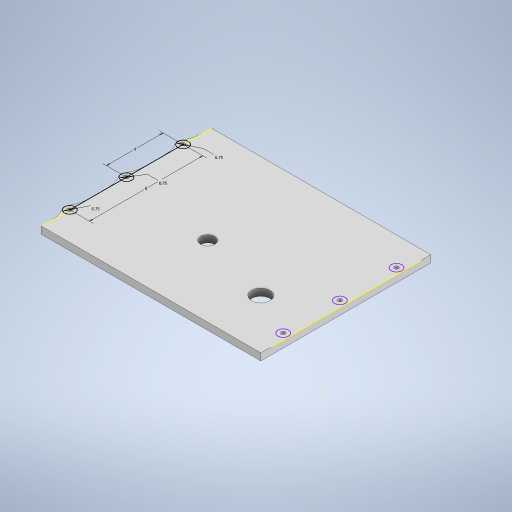
# Autodesk Inventor part: chassis_cap
Saved by Autodesk Inventor 2023 (Build 270158000, 158)
## iProperties
Created: 2023-05-04
Part Number: chassis_cap
Material: Generic
Document SubType Name: Modeling
Designer: user
Density: 1 g/cm^3
Appearance: Default
Author: user
Autodesk Inventor part; units mm, degrees
ref_plane "YZ Plane" through (0, 0, 0) normal (1, 0, 0) x (0, 1, 0)
ref_plane "XZ Plane" through (0, 0, 0) normal (0, 1, 0) x (-1, 0, 0)
ref_plane "XY Plane" through (0, 0, 0) normal (0, 0, 1) x (1, 0, 0)
sketch "Sketch2" plane through (0, 0, 0) normal (0, 1, 0) x (-1, 0, 0)
  line L0 (0, 0) -> (200, 0)
  line L1 (200, 0) -> (200, -120)
  line L2 (200, -120) -> (0, -120)
  line L3 (0, -120) -> (0, 0)
  dimension "d0" = 200
  dimension "d1" = 120
  constraints: 8 end point, 2 parallel, 1 horizontal, 1 perpendicular
  measures "d0" distance of L1.end L2.end
  measures "d1" distance of L0.end L1.end
extrude "Extrusion1" add sketch "Sketch2" along normal blind 50
sketch "Sketch3" plane through (0, 50, 0) normal (0, 1, 0) x (1, 0, 0)
  line L0 (0, 120) -> (-200, 120) projected
  line L1 (0, 120) -> (0, 113)
  line L2 (0, 0) -> (0, 120) projected
  line L3 (-200, 0) -> (0, 0) projected
  line L4 (0, 0) -> (0, 7)
  line L5 (0, 7) -> (-45, 7)
  line L6 (-45, 7) -> (-45, 113)
  line L7 (-45, 113) -> (0, 113)
  line L8 (0, 113) -> (0, 7)
  dimension "d4" = 7
  dimension "d5" = 7
  dimension "d6" = 45
  constraints: 12 end point, 2 parallel, 2 point on line, 1 horizontal, 1 perpendicular
  measures "d4" distance of L0.start L1.end
  measures "d5" distance of L2.start L4.end
  measures "d6" distance of L6.end L7.end
extrude "Extrusion2" cut sketch "Sketch3" against normal blind 50
sketch "Sketch6" plane through (-200, 0, 0) normal (0, 0, 1) x (1, 0, 0)
  line L0 (200, 0) -> (200, 50) projected
  line L1 (200, 0) -> (205, 0)
  line L2 (205, 0) -> (205, 50)
  line L3 (205, 50) -> (200, 50)
  line L4 (200, 50) -> (200, 0)
  dimension "d42" = 5
  constraints: 8 end point, 2 parallel, 1 horizontal, 1 perpendicular
  measures "d42" distance of L3.end L2.end
extrude "Extrusion4" add sketch "Sketch6" against normal blind 7
sketch "Sketch7" plane through (0, 0, -120) normal (0, 0, -1) x (-1, 0, 0)
  line L0 (45, 50) -> (0, 50) projected
  line L1 (200, 0) -> (-5, 0) projected
  line L2 (0, 50) -> (-5, 50)
  line L3 (-5, 50) -> (-5, 0)
  line L4 (-5, 0) -> (0, 0)
  line L5 (0, 0) -> (0, 50)
  constraints: 8 end point, 2 parallel, 1 horizontal, 1 perpendicular
extrude "Extrusion5" add sketch "Sketch7" against normal blind 7
sketch "Sketch8" plane through (0, 0, 0) normal (0, -1, 0) x (1, 0, 0)
  line L0 (-200, -120) -> (-200, 0) projected
  line L1 (-200, 0) -> (5, 0) projected
  line L2 (-200, 0) -> (-195, 0)
  line L3 (-45, -113) -> (-45, -7) projected
  line L4 (-200, -120) -> (5, -120) projected
  line L5 (-45, -113) -> (-52, -113)
  line L6 (-52, -113) -> (-52, -120)
  line L7 (-52, -120) -> (-45, -120)
  line L8 (-45, -120) -> (-45, -113)
  line L9 (-45, -7) -> (5, -7) projected
  line L10 (-45, -7) -> (-52, -7)
  line L11 (-52, -7) -> (-52, 0)
  line L12 (-52, 0) -> (-45, 0)
  line L13 (-45, 0) -> (-45, -7)
  line L14 (-200, 0) -> (-193, 0)
  line L15 (-193, 0) -> (-193, -7)
  line L16 (-193, -7) -> (-200, -7)
  line L17 (-200, -7) -> (-200, 0)
  line L18 (-200, -120) -> (-193, -120)
  line L19 (-193, -120) -> (-193, -113)
  line L20 (-193, -113) -> (-200, -113)
  line L21 (-200, -113) -> (-200, -120)
  line L22 (-193, -113) -> (-52, -113)
  line L23 (-52, -113) -> (-52, -7)
  line L24 (-52, -7) -> (-193, -7)
  line L25 (-193, -7) -> (-193, -113)
  point P0 (0, 0)
  dimension "d51" = 7
  dimension "d52" = 7
  dimension "d53" = 7
  dimension "d54" = 7
  dimension "d55" = 7
  dimension "d56" = 7
  dimension "d57" = 7
  constraints: 42 end point, 10 parallel, 6 horizontal, 5 perpendicular, 1 point on line
  measures "d51" distance of L7.end L6.end
  measures "d52" distance of L11.end L12.end
  measures "d53" distance of L10.end L11.end
  measures "d54" distance of L15.end L16.end
  measures "d55" distance of L14.end L15.end
  measures "d56" distance of L20.end L19.end
  measures "d57" distance of L19.end L18.end
extrude "Extrusion6" cut sketch "Sketch8" against normal blind 45 contours L25 L24 L23 L22
sketch "Sketch9" plane through (-45, 50, -7) normal (1, 0, 0) x (0, 0, -1)
  line L0 (106, -50) -> (0, -50) projected
  line L1 (53, -50) -> (53, 0)
  line L2 (0, 0) -> (106, 0) projected
  line L3 (53, -25) -> (106, -25)
  line L4 (106, -25) -> (84, -25)
  line L5 (84, -25) -> (84, -15)
  line L6 (84, -25) -> (84, -35)
  line L7 (84, -35) -> (72, -35)
  line L8 (72, -35) -> (72, -15)
  line L9 (72, -15) -> (84, -15)
  line L10 (84, -15) -> (84, -35)
  line L11 (106, 0) -> (0, 0)
  line L12 (53, -25) -> (0, -25)
  line L13 (0, -25) -> (22, -25)
  line L14 (106, -25) -> (86, -25)
  line L15 (86, -25) -> (69.9067, -25)
  line L16 (69.9067, -25) -> (69.9067, -38.406)
  line L17 (69.9067, -38.406) -> (86, -38.406)
  line L18 (86, -38.406) -> (86, -25)
  line L19 (86, -25) -> (69.9067, -25)
  line L20 (69.9067, -25) -> (69.9067, -11.59)
  line L21 (69.9067, -11.59) -> (86, -11.59)
  line L22 (86, -11.59) -> (86, -25)
  line L23 (53, -25) -> (0, -25)
  line L24 (0, -25) -> (22, -25)
  line L25 (22, -25) -> (22, -15)
  line L26 (22, -25) -> (22, -35)
  line L27 (22, -35) -> (34, -35)
  line L28 (34, -35) -> (34, -15)
  line L29 (34, -15) -> (22, -15)
  line L30 (22, -15) -> (22, -35)
  line L31 (0, -25) -> (20, -25)
  line L32 (20, -25) -> (36.0933, -25)
  line L33 (36.0933, -25) -> (36.0933, -38.406)
  line L34 (36.0933, -38.406) -> (20, -38.406)
  line L35 (20, -38.406) -> (20, -25)
  line L36 (20, -25) -> (36.0933, -25)
  line L37 (36.0933, -25) -> (36.0933, -11.59)
  line L38 (36.0933, -11.59) -> (20, -11.59)
  line L39 (20, -11.59) -> (20, -25)
  point P0 (-7, -50)
  dimension "d60" = 22
  dimension "d61" = 10
  dimension "d62" = 10
  dimension "d63" = 12
  dimension "d66" = 20
  dimension "d67" = 13.41
  dimension "d68" = 13.4061
  constraints: 76 end point, 16 symmetric about line, 6 parallel, 5 perpendicular, 5 point on line, 4 horizontal, 3 midpoint
  measures "d60" distance of L3.end L4.end
  measures "d61" distance of L4.end L5.end
  measures "d62" distance of L4.end L6.end
  measures "d63" distance of L8.end L9.end
  measures "d66" distance of L3.end L14.end
  measures "d67" distance of L19.end L20.end
  measures "d68" distance of L15.end L16.end
extrude "Extrusion8" cut sketch "Sketch9" against normal blind 10
sketch "Sketch10" plane through (0, 45, 0) normal (0, -1, 0) x (1, 0, 0)
  line L0 (-193, -113) -> (-193, -7) projected
  line L1 (-193, -60) -> (-148, -60)
  line L2 (-148, -7) -> (-143, -7)
  line L3 (-143, -7) -> (-143, -95.0021)
  line L4 (-143, -95.0021) -> (-148, -95.0021)
  line L5 (-148, -95.0021) -> (-148, -7)
  point P0 (0, 0)
  dimension "d71" = 45
  dimension "d72" = 5
  constraints: 10 end point, 2 horizontal, 2 parallel, 1 midpoint, 1 perpendicular
  measures "d71" distance of L1.start L1.end
  measures "d72" distance of L3.end L4.end
extrude "Extrusion9" add sketch "Sketch10" along normal blind 40
sketch "Sketch11" plane through (0, 0, 0) normal (0, -1, 0) x (1, 0, 0)
  line L0 (-148, -7) -> (-148, -95.0021) projected
  line L1 (-148, -95.0021) -> (-148, -114.483)
  line L2 (-52, -113) -> (-193, -113) projected
  line L3 (-193, -113) -> (-148, -113)
  line L4 (-148, -113) -> (-148, -117)
  line L5 (-148, -117) -> (-193, -117)
  line L6 (-193, -117) -> (-193, -113)
  line L7 (-193, -7) -> (-52, -7) projected
  line L8 (-193, -7) -> (-148, -7)
  line L9 (-148, -7) -> (-148, -3)
  line L10 (-148, -3) -> (-193, -3)
  line L11 (-193, -3) -> (-193, -7)
  point P0 (0, 0)
  dimension "d75" = 4
  dimension "d76" = 4
  constraints: 18 end point, 4 parallel, 2 horizontal, 2 perpendicular, 1 point on line, 1 vertical
  measures "d75" distance of L3.end L4.end
  measures "d76" distance of L9.end L8.end
extrude "Extrusion10" cut sketch "Sketch11" against normal blind 45
sketch "Sketch12" plane through (-52, 0, -113) normal (0, 0, 1) x (1, 0, 0)
  line L0 (0, 0) -> (0, 45) projected
  line L1 (0, 45) -> (-91, 45)
  line L2 (-91, 45) -> (-91, 0)
  line L3 (-91, 0) -> (0, 0)
  line L4 (0, 0) -> (0, 45)
  line L5 (-69.4543, 22.5) -> (-21.0513, 22.5) construction
  line L6 (-69.4543, 10.4971) -> (-21.0513, 10.4971)
  line L7 (-21.0513, 34.5029) -> (-69.4543, 34.5029)
  arc A0 (-69.4543, 34.5029) -> (-69.4543, 10.4971) centre (-69.4543, 22.5) ccw
  arc A1 (-21.0513, 10.4971) -> (-21.0513, 34.5029) centre (-21.0513, 22.5) ccw
  point P0 (52, 0)
  point P1 (-45.2528, 22.5)
  constraints: 16 end point, 4 point on circle, 4 tangent, 3 parallel, 2 centre point, 2 horizontal, 1 midpoint, 1 perpendicular
extrude "Extrusion11" cut sketch "Sketch12" along normal mid plane 2000 contours A0 L7 A1 L6
sketch "Sketch13" plane through (0, 0, 0) normal (0, -1, 0) x (1, 0, 0)
  line L0 (-200, -120) -> (-200, 0) projected
  line L1 (-200, -60) -> (-200, -100)
  line L2 (-200, -100) -> (-200, -20)
  circle A0 centre (-200, -20) radius 3.75
  circle A1 centre (-200, -60) radius 3.75
  circle A2 centre (-200, -100) radius 3.75
  circle A3 centre (-49.267, -60) radius 3.75
  circle A4 centre (-49.267, -100) radius 3.75
  circle A5 centre (-49.267, -20) radius 3.75
  line L3 (-45, -113) -> (-45, -7) projected
  point P0 (0, 0)
  dimension "d81" = 40
  dimension "d82" = 80
  dimension "d83" = 7.5
  dimension "d84" = 7.5
  dimension "d85" = 7.5
  constraints: 6 centre point, 4 end point, 3 coincident, 2 point on line, 1 midpoint
  measures "d81" distance of L1.start L1.end
  measures "d82" distance of L1.end L2.end
  measures "d83" diameter of A0
  measures "d84" diameter of A1
  measures "d85" diameter of A2
extrude "Extrusion12" add sketch "Sketch13" against normal blind 17.5 contours A2 L0 | L0 A2 | A1 L0 | L0 A1 | A0 L0 | L0 A0 | A3
extrude "Extrusion13" add sketch "Sketch13" against normal blind 17.5 contours A3 | A4 | A5
sketch "Sketch16" plane through (0, 0, 0) normal (0, -1, 0) x (1, 0, 0)
  arc A0 (-200, -16.25) -> (-200, -23.75) centre (-200, -20) ccw projected
  circle A1 centre (-200, -20) radius 1.5
  line L0 (-200, -120) -> (-200, 0) projected
  circle A2 centre (-200, -60) radius 1.5
  circle A3 centre (-200, -99.9997) radius 1.5
  circle A4 centre (-49.3006, -99.9997) radius 1.5
  circle A5 centre (-49.3006, -60) radius 1.5
  circle A6 centre (-49.3006, -20) radius 1.5
  point P0 (0, 0)
  dimension "d90" = 3
  dimension "d91" = 3
  dimension "d92" = 3
  dimension "d93" = 3
  dimension "d94" = 3
  dimension "d95" = 3
  constraints: 6 centre point, 1 coincident, 1 midpoint
  measures "d90" diameter of A1
  measures "d91" diameter of A2
  measures "d92" diameter of A3
  measures "d93" diameter of A4
  measures "d94" diameter of A5
  measures "d95" diameter of A6
extrude "Extrusion14" cut sketch "Sketch16" along normal mid plane 15 contours L0 A1 | A1 L0 | A3 L0 | L0 A3 | A2 L0 | L0 A2 | A4 | A5 | A6
fillet "Fillet1" radius 3.5875 3 edges at (-203.75, 17.5, -60) (-203.75, 17.5, -100) (-203.75, 17.5, -20)
fillet "Fillet2" radius 2 3 edges at (-53.017, 17.5, -100) (-53.017, 17.5, -60) (-53.017, 17.5, -20)
sketch "Sketch17" plane through (0, 45, 0) normal (0, -1, 0) x (1, 0, 0)
  line L0 (-148, -7) -> (-52, -7) projected
  line L1 (-142.7275, -7) -> (-52, -7)
  line L2 (-52, -7) -> (-52, -113)
  line L3 (-52, -113) -> (-142.7275, -113)
  circle A0 centre (-49.3006, -60) radius 1.5 projected
  line L4 (-49.3006, -60) -> (-200.2165, -60)
  line L5 (-121.4543, -7) -> (-73.0513, -7) projected
  line L6 (-97.2528, -7) -> (-64.7528, -7)
  line L7 (-64.7528, -7) -> (-97.2528, -7)
  line L8 (-97.2528, -7) -> (-129.7528, -7)
  line L9 (-148, -7) -> (-143, -7) projected
  line L10 (-143, -7) -> (-129.7528, -7)
  line L11 (-143, -7) -> (-64.7528, -7)
  circle A1 centre (-64.7528, -101.7496) radius 2
  circle A2 centre (-64.7528, -18.25) radius 2
  circle A3 centre (-129.7528, -18.25) radius 2
  circle A4 centre (-129.7528, -101.7496) radius 2
  point P0 (0, 0)
  dimension "d105" = 32.5
  dimension "d106" = 32.5
  dimension "d107" = 32.5
  dimension "d108" = 4
  dimension "d109" = 4
  dimension "d110" = 4
  dimension "d111" = 4
  constraints: 18 end point, 4 centre point, 4 horizontal, 3 point on line, 1 coincident, 1 collinear, 1 midpoint, 1 parallel, 1 perpendicular
  measures "d105" distance of L6.start L6.end
  measures "d106" distance of L6.end L6.start
  measures "d107" distance of L6.start L8.end
  measures "d108" diameter of A1
  measures "d109" diameter of A2
  measures "d110" diameter of A3
  measures "d111" diameter of A4
extrude "Extrusion15" cut sketch "Sketch17" against normal blind 15 contours A1 | A2 | A3 | A4
fillet "Fillet3" radius 19.4625 15 edges at (-200, 16.4492, -17.3007) (-200, 16.4492, -22.6993) (-200, 17.5, -20) (-200, 6.9562, -16.25) (-200, 6.9562, -23.75) (-200, 16.4492, -62.6992) (-200, 16.4492, -57.3008) (-200, 17.5, -60) (-200, 6.9562, -63.75) (-200, 6.9562, -56.25) (-200, 16.4492, -102.6993) (-200, 16.4492, -97.3007) (-200, 17.5, -100) (-200, 6.9562, -103.75) (-200, 6.9562, -96.25)
sketch "Sketch18" plane through (-200, 0, -120) normal (0, 0, -1) x (-1, 0, 0)
  line L0 (-155, 50) -> (-155, 0) projected
  line L1 (-155, 0) -> (-155, 50)
  circle A0 centre (0, 0) radius 11.05
  circle A1 centre (-15.5, 15.5) radius 1.75
  circle A2 centre (15.5, 15.5) radius 1.75
  circle A3 centre (15.5, -15.5) radius 1.75
  circle A4 centre (-15.5, -15.5) radius 1.75
  circle A5 centre (0, 0) radius 11.05
  circle A6 centre (-15.5, 15.5) radius 1.75
  circle A7 centre (15.5, 15.5) radius 1.75
  circle A8 centre (15.5, -15.5) radius 1.75
  circle A9 centre (-15.5, -15.5) radius 1.75
  circle A10 centre (0, 0) radius 11.05
  circle A11 centre (-15.5, 15.5) radius 1.75
  circle A12 centre (15.5, 15.5) radius 1.75
  circle A13 centre (15.5, -15.5) radius 1.75
  circle A14 centre (-15.5, -15.5) radius 1.75
  line L2 (-205, 0) -> (-205, 50) projected
  line L3 (-155, 0) -> (-205, 0)
  line L4 (-205, 0) -> (-205, 50)
  line L5 (-205, 50) -> (-155, 50)
  line L6 (-155, 50) -> (-155, 0)
  circle A15 centre (-180, 25) radius 11.5
  line L7 (-180, 25) -> (-164.5, 25)
  line L8 (-164.5, 25) -> (-164.5, 50)
  line L9 (-205, 50) -> (-155, 50) projected
  line L10 (-205, 0) -> (0, 0) projected
  line L11 (-164.5, 0) -> (-164.5, 25)
  line L12 (-180, 25) -> (-195.5, 25)
  line L13 (-195.5, 25) -> (-195.5, 50)
  line L14 (-195.5, 0) -> (-195.5, 25)
  line L15 (-180, 25) -> (-180, 9.5)
  line L16 (-180, 25) -> (-180, 40.5)
  line L17 (-180, 40.5) -> (-164.5, 40.5)
  line L18 (-180, 40.5) -> (-195.5, 40.5)
  line L19 (-180, 9.5) -> (-164.5, 9.5)
  line L20 (-180, 9.5) -> (-195.5, 9.5)
  circle A16 centre (-164.5, 9.5) radius 2.5
  circle A17 centre (-164.5, 40.5) radius 2.5
  circle A18 centre (-195.5, 40.5) radius 2.5
  circle A19 centre (-195.5, 9.5) radius 2.5
  point P0 (-200, 0)
  dimension "d115" = 22.1
  dimension "d116" = 31
  dimension "d117" = 31
  dimension "d118" = 31
  dimension "d119" = 31
  dimension "d120" = 3.5
  dimension "d121" = 3.5
  dimension "d122" = 3.5
  dimension "d123" = 3.5
  dimension "d124" = 15.5
  dimension "d125" = 15.5
  dimension "d126" = 15.5
  dimension "d127" = 15.5
  dimension "d128" = 22.1
  dimension "d129" = 31
  dimension "d130" = 31
  dimension "d131" = 31
  dimension "d132" = 31
  dimension "d133" = 3.5
  dimension "d134" = 3.5
  dimension "d135" = 3.5
  dimension "d136" = 3.5
  dimension "d137" = 15.5
  dimension "d138" = 15.5
  dimension "d139" = 15.5
  dimension "d140" = 15.5
  dimension "d141" = 22.1
  dimension "d142" = 31
  dimension "d143" = 31
  dimension "d144" = 31
  dimension "d145" = 31
  dimension "d146" = 3.5
  dimension "d147" = 3.5
  dimension "d148" = 3.5
  dimension "d149" = 3.5
  dimension "d150" = 15.5
  dimension "d151" = 15.5
  dimension "d152" = 15.5
  dimension "d153" = 15.5
  dimension "d154" = 23
  dimension "d156" = 15.5
  dimension "d157" = 15.5
  dimension "d158" = 5
  dimension "d159" = 5
  dimension "d160" = 5
  dimension "d161" = 5
  constraints: 34 end point, 20 centre point, 10 point on line, 7 coincident, 6 perpendicular, 3 equal length, 2 horizontal, 1 vertical
  measures "d115" diameter of A0
  measures "d116" distance of A2.centre A1.centre
  measures "d117" distance of A3.centre A2.centre
  measures "d118" distance of A1.centre A4.centre
  measures "d119" distance of A3.centre A4.centre
  measures "d120" diameter of A1
  measures "d121" diameter of A2
  measures "d122" diameter of A4
  measures "d123" diameter of A3
  measures "d124" horizontal distance of A1.centre L10.end
  measures "d125" horizontal distance of L10.end A1.centre
  measures "d126" horizontal distance of L10.end A3.centre
  measures "d127" horizontal distance of L10.end A3.centre
  measures "d128" diameter of A5
  measures "d129" distance of A7.centre A6.centre
  measures "d130" distance of A8.centre A7.centre
  measures "d131" distance of A6.centre A9.centre
  measures "d132" distance of A8.centre A9.centre
  measures "d133" diameter of A6
  measures "d134" diameter of A7
  measures "d135" diameter of A9
  measures "d136" diameter of A8
  measures "d137" horizontal distance of A6.centre point (0, 0)
  measures "d138" horizontal distance of point (0, 0) A6.centre
  measures "d139" horizontal distance of point (0, 0) A8.centre
  measures "d140" horizontal distance of point (0, 0) A8.centre
  measures "d141" diameter of A10
  measures "d142" distance of A12.centre A11.centre
  measures "d143" distance of A13.centre A12.centre
  measures "d144" distance of A11.centre A14.centre
  measures "d145" distance of A13.centre A14.centre
  measures "d146" diameter of A11
  measures "d147" diameter of A12
  measures "d148" diameter of A14
  measures "d149" diameter of A13
  measures "d150" horizontal distance of A11.centre point (0, 0)
  measures "d151" horizontal distance of point (0, 0) A11.centre
  measures "d152" horizontal distance of point (0, 0) A13.centre
  measures "d153" horizontal distance of point (0, 0) A13.centre
  measures "d154" diameter of A15
  measures "d156" distance of L7.start L15.end
  measures "d157" distance of L7.start L16.end
  measures "d158" diameter of A16
  measures "d159" diameter of A17
  measures "d160" diameter of A18
  measures "d161" diameter of A19
extrude "Extrusion16" cut sketch "Sketch18" against normal blind 2000 contours A17 L8 | L8 L17 A17 | A16 L19 L11 | L11 A16 | A18 L18 L13 | L13 A18 | L8 A17 L17 | A19 L14 | L14 L20 A19 | L19 A16 L11 | L18 A18 L13 | L14 A19 L20 | L16 L12 A15 | A15 L7 L16 | L15 L7 A15 | A15 L12 L15
sketch "Sketch19" plane through (0, 45, 0) normal (0, -1, 0) x (1, 0, 0)
  circle A0 centre (-129.7528, -101.7496) radius 2 projected
  circle A1 centre (-129.7528, -18.25) radius 2 projected
  line L0 (-129.7528, -101.7496) -> (-129.7528, -18.25)
  circle A2 centre (-64.7528, -18.25) radius 2 projected
  line L1 (-129.7528, -18.25) -> (-64.7528, -18.25)
  circle A3 centre (-64.7528, -101.7496) radius 2 projected
  line L2 (-64.7528, -18.25) -> (-64.7528, -101.7496)
  line L3 (-64.7528, -101.7496) -> (-129.7528, -101.7496)
  line L4 (-87.014, -168.9687) -> (-85.0378, -168.9687)
  circle A4 centre (-49.3006, -20) radius 1.5 projected
  circle A5 centre (-49.3006, -20) radius 1.5
  circle A6 centre (-49.3006, -59.9998) radius 1.5002
  circle A7 centre (-49.3006, -99.9997) radius 1.5 projected
  circle A8 centre (-49.3006, -99.9997) radius 1.5
  line L5 (-200, -120) -> (-200, 0) projected
  circle A9 centre (-200, -99.9997) radius 1.5
  circle A10 centre (-200, -60) radius 1.5 projected
  circle A11 centre (-200, -60) radius 1.5
  circle A12 centre (-200, -20) radius 1.5
  point P0 (0, 0)
  constraints: 10 end point, 6 centre point, 3 coincident, 3 perpendicular, 1 horizontal, 1 point on line
extrude "Extrusion17" add sketch "Sketch19" along normal blind 100 contours A4 | A6 | A7 | A9 L5 | L5 A9 | A10 L5 | L5 A10 | A12 L5 | L5 A12
sketch "Sketch20" plane through (0, 0, 0) normal (0, -1, 0) x (1, 0, 0)
  line L0 (5, -120) -> (-200, -120) projected
  line L1 (-45, 0) -> (-200, 0)
  line L2 (-200, 0) -> (-200, -120)
  line L3 (-200, -120) -> (-45, -120)
  line L4 (-45, -120) -> (-45, 0)
  line L5 (-200, -61.5) -> (-200, -58.5) projected
  circle A0 centre (-200, -60) radius 3.7248
  line L6 (-200, -101.4997) -> (-200, -98.4997) projected
  circle A1 centre (-200, -99.9997) radius 3.7458
  line L7 (-200, -21.5) -> (-200, -18.5) projected
  circle A2 centre (-200, -20) radius 3.7312
  point P0 (0, 0)
  point P1 (-200, -16.2688)
  point P2 (-200, -23.7312)
  point P3 (-200, -56.2752)
  point P4 (-200, -63.7248)
  point P5 (-200, -96.2539)
  point P6 (-200, -103.7454)
  constraints: 8 end point, 3 centre point, 3 midpoint, 2 parallel, 1 horizontal, 1 perpendicular
extrude "Extrusion18" add sketch "Sketch20" along normal blind 5
fillet "Fillet4" radius 19.4625 6 edges at (-200, -2.5, -96.2539) (-200, -2.5, -103.7454) (-200, -2.5, -63.7248) (-200, -2.5, -56.2752) (-200, -2.5, -16.2688) (-200, -2.5, -23.7312)
sketch "Sketch21" plane through (0, -5, 0) normal (0, -1, 0) x (1, 0, 0)
  point P0 (0, 0)
sketch "Sketch22" plane through (0, 50, 0) normal (0, 1, 0) x (1, 0, 0)
  line L0 (-218.9045, 160.531) -> (29.7585, 160.531)
  line L1 (29.7585, 160.531) -> (29.7585, -28.8143)
  line L2 (29.7585, -28.8143) -> (-218.9045, -28.8143)
  line L3 (-218.9045, -28.8143) -> (-218.9045, 160.531)
  point P0 (0, 0)
  constraints: 8 end point, 2 parallel, 1 horizontal, 1 perpendicular
extrude "Extrusion19" cut sketch "Sketch22" against normal blind 50
sketch "Sketch24" plane through (0, -5, 0) normal (0, -1, 0) x (1, 0, 0)
  circle A0 centre (-49.3006, -20) radius 1.5 projected
  circle A1 centre (-49.3006, -20) radius 1.5
  circle A2 centre (-49.3006, -59.9998) radius 1.5002 projected
  circle A3 centre (-49.3006, -59.9998) radius 1.5002
  circle A4 centre (-49.3006, -99.9997) radius 1.5 projected
  circle A5 centre (-49.3006, -99.9997) radius 1.5
  circle A6 centre (-200, -99.9997) radius 1.5 projected
  circle A7 centre (-200, -99.9997) radius 1.5
  circle A8 centre (-200, -60) radius 1.5 projected
  circle A9 centre (-200, -60) radius 1.5
  circle A10 centre (-200, -20) radius 1.5 projected
  circle A11 centre (-200, -20) radius 1.5
  point P0 (0, 0)
  constraints: 6 centre point, 6 coincident
extrude "Extrusion20" cut sketch "Sketch24" along normal mid plane 500
sketch "Sketch25" plane through (0, -5, 0) normal (0, -1, 0) x (1, 0, 0)
  line L0 (-45, -120) -> (-45, 0) projected
  line L1 (-45, 0) -> (-132.5, 0)
  line L2 (-132.5, 0) -> (-132.5, -50)
  line L3 (-132.5, -50) -> (-45, -50)
  line L4 (-45, -50) -> (-45, 0)
  circle A0 centre (-132.5, -50) radius 5
  line L5 (-45, 0) -> (-200, 0) projected
  line L6 (-45, 0) -> (-80, 0)
  line L7 (-80, 0) -> (-80, -35)
  line L8 (-80, -35) -> (-45, -35)
  line L9 (-45, -35) -> (-45, 0)
  circle A1 centre (-80, -35) radius 6.5
  point P0 (0, 0)
  dimension "d181" = 87.5
  dimension "d182" = 50
  dimension "d183" = 10
  dimension "d184" = 35
  dimension "d185" = 35
  dimension "d186" = 13
  constraints: 16 end point, 4 parallel, 2 centre point, 2 coincident, 2 horizontal, 2 perpendicular
  measures "d181" distance of L3.end L2.end
  measures "d182" distance of L2.end L1.end
  measures "d183" diameter of A0
  measures "d184" distance of L8.end L7.end
  measures "d185" distance of L7.end L6.end
  measures "d186" diameter of A1
extrude "Extrusion21" cut sketch "Sketch25" against normal blind 500 contours A0 L2 L3 | L3 L2 A0 | A1 L7 L8 | L8 L7 A1
equation "\"d69\" = d62"
body "Solid1"
